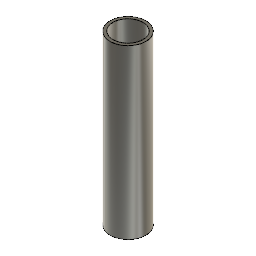
pen_part2 (Autodesk Fusion 360 design; units mm, degrees)
Autodesk Fusion 360 part; units mm, degrees
cylinder "CylinderPrimitive1" add diameter 15 height 70 placed x (1, 0, 0) y (0, 1, 0) z (0, 0, 1) at (0, 0, 0)
sketch "Sketch2" plane through (0, 0, 70) normal (0, 0, 1) x (-1, 0, 0)
  circle A0 centre (0, 0) radius 7.5
  circle A1 centre (0, 0) radius 6.25
  dimension "d3" = 12.5
  constraint concentric A0 A1
  measures "d3" diameter of A1
extrude "Extrude1" cut sketch "Sketch2" against normal blind 65 contours A1
hole "Hole1" at (-0.0348, -0.2802, 5) direction (0, 0, -1) diameter 1 depth 5 tip angle 180
